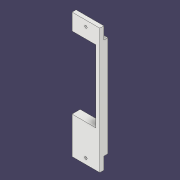
# Autodesk Inventor part: BP005
Saved by Autodesk Inventor 2017 SP1 (Build 210196100, 196)
## iProperties
Created: 2018-01-07
Part Number: BP005
Material: ABS Plastic
Document SubType Name: Modeling
Designer: Zach
Density: 1.06 g/cm^3
Appearance: CR White
Author: Zach
Autodesk Inventor part; units mm, degrees
ref_plane "YZ Plane" through (0, 0, 0) normal (1, 0, 0) x (0, 1, 0)
ref_plane "XZ Plane" through (0, 0, 0) normal (0, 1, 0) x (-1, 0, 0)
ref_plane "XY Plane" through (0, 0, 0) normal (0, 0, 1) x (1, 0, 0)
sketch "Sketch1" plane through (0, 0, 0) normal (0, 0, 1) x (1, 0, 0)
  line L0 (0, 0) -> (34, 0)
  line L1 (34, 0) -> (34, 153)
  line L2 (34, 153) -> (0, 153)
  line L3 (0, 153) -> (0, 0)
  circle A0 centre (17, 7) radius 1.5
  circle A1 centre (17, 146) radius 1.5
  point P0 (17, 153)
  point P1 (17, 0)
  dimension "d0" = 34
  dimension "d1" = 153
  dimension "d2" = 3
  dimension "d4" = 7
  dimension "d5" = 3
  dimension "d6" = 7
  constraints: 8 end point, 2 centre point, 2 midpoint, 2 parallel, 2 vertical alignment, 1 horizontal, 1 perpendicular
  measures "d0" distance of L2.end L1.end
  measures "d1" distance of L1.end L0.end
  measures "d2" diameter of A0
  measures "d4" distance from line of L0 A0.centre
  measures "d5" diameter of A1
  measures "d6" distance from line of L2 A1.centre
extrude "Extrusion1" add sketch "Sketch1" along normal blind 5
sketch "Sketch2" plane through (0, 0, 0) normal (0, 0, -1) x (-1, 0, 0)
  line L0 (0, 153) -> (0, 0) projected
  line L1 (0, 138) -> (-34, 138)
  line L2 (-34, 138) -> (-34, 15)
  line L3 (-34, 15) -> (0, 15)
  line L4 (0, 15) -> (0, 138)
  line L5 (-34, 0) -> (-34, 153) projected
  point P0 (0, 76.5)
  dimension "d10" = 123
  constraints: 8 end point, 2 midpoint, 2 parallel, 2 point on line, 1 horizontal, 1 perpendicular
  measures "d10" distance of L2.end L1.end
extrude "Extrusion2" add sketch "Sketch2" along normal blind 5
sketch "Sketch7" plane through (0, 0, 5) normal (0, 0, 1) x (1, 0, 0)
  line L0 (29, 133) -> (0, 133)
  line L1 (0, 133) -> (0, 45)
  line L2 (0, 45) -> (29, 45)
  line L3 (29, 45) -> (29, 133)
  line L4 (34, 0) -> (34, 153) projected
  line L5 (34, 153) -> (0, 153) projected
  line L6 (0, 15) -> (34, 15) projected
  line L7 (34, 138) -> (0, 138) projected
  line L8 (0, 153) -> (0, 0) projected
  point P0 (29, 89)
  point P1 (17, 153)
  dimension "d33" = 30
  dimension "d34" = 5
  dimension "d35" = 5
  constraints: 8 end point, 2 midpoint, 2 parallel, 1 horizontal, 1 perpendicular, 1 point on line
  measures "d33" distance between parallel lines of L6 L2
  measures "d34" distance between parallel lines of L7 L0
  measures "d35" distance between parallel lines of L4 L3
extrude "Extrusion5" cut sketch "Sketch7" against normal through all contours L3 L2 L1 L0
body "Solid1"
